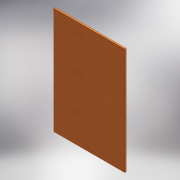
# Autodesk Inventor part: puerta_lavaplatos
Saved by Autodesk Inventor 2016 (Build 200138000, 138)
## iProperties
Created: 2015-11-25
Part Number: puerta_lavaplatos
Material: Generic
Document SubType Name: Modeling
Designer: Daniela
Density: 1 g/cm^3
Appearance: White
Author: Daniela
Autodesk Inventor part; units mm, degrees
ref_plane "YZ Plane" through (0, 0, 0) normal (1, 0, 0) x (0, 1, 0)
ref_plane "XZ Plane" through (0, 0, 0) normal (0, 1, 0) x (-1, 0, 0)
ref_plane "XY Plane" through (0, 0, 0) normal (0, 0, 1) x (1, 0, 0)
sketch "Sketch8" plane through (0, 0, 0) normal (0, 1, 0) x (-1, 0, 0)
  line L0 (0, 0) -> (10, 0)
  line L1 (0, 0) -> (0, 70)
  line L2 (0, 70) -> (20, 70)
  line L3 (20, 70) -> (550, 70)
  line L4 (550, 70) -> (550, 870)
  line L5 (550, 870) -> (20, 870)
  line L6 (20, 870) -> (20, 70)
  line L7 (550, 790) -> (20, 790) construction
  circle A0 centre (500, 843) radius 3
  line L8 (500, 843) -> (500, 743)
  circle A1 centre (500, 743) radius 3
  dimension "espesor" = 10
  dimension "d38" = 70
  dimension "d39" = 20
  dimension "ancho_m" = 530
  dimension "h_inf" = 800
  dimension "d42" = 80
  dimension "d43" = 6
  dimension "d44" = 50
  dimension "d45" = 50
  dimension "d48" = 100
  dimension "d49" = 6
  constraints: 18 end point, 3 perpendicular, 2 centre point, 2 horizontal, 2 parallel, 2 point on line, 2 vertical, 1 coincident
  measures "espesor" distance of L0.start L0.end
  measures "d38" distance of L0.start L1.end
  measures "d39" distance of L1.end L2.end
  measures "ancho_m" distance of L5.end L4.end
  measures "h_inf" distance of L4.end L3.end
  measures "d42" distance between parallel lines of L5 L7
  measures "d43" diameter of A0
  measures "d44" distance edge to line of A0 L7
  measures "d45" distance from line of L4 L8.start
  measures "d48" distance of L8.start L8.end
  measures "d49" diameter of A1
extrude "Extrusion8" add sketch "Sketch8" along normal blind 10
equation "\"d39\" = 2 * espesor"
equation "\"d42\" = 0.1 * h_inf"
equation "\"d46\" = espesor"
body "Solid2"
